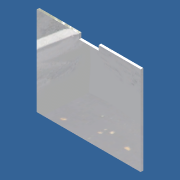
# Autodesk Inventor part: side panel for hinge
Saved by Autodesk Inventor 2012 (Build 160160000, 160)
## iProperties
Created: 2012-02-06
Part Number: side panel for hinge
Material: Default
Document SubType Name: Modeling
Designer: Allison Garza
Density: 1 g/cm^3
Author: Allison Garza
Autodesk Inventor part; units mm, degrees
ref_plane "YZ Plane" through (0, 0, 0) normal (1, 0, 0) x (0, 1, 0)
ref_plane "XZ Plane" through (0, 0, 0) normal (0, 1, 0) x (-1, 0, 0)
ref_plane "XY Plane" through (0, 0, 0) normal (0, 0, 1) x (1, 0, 0)
sketch "Sketch1" plane through (0, 0, 0) normal (0, 0, 1) x (1, 0, 0)
  line L0 (-13.9496, 17.395) -> (119.4004, 17.395)
  line L1 (119.4004, 17.395) -> (119.4004, -96.905)
  line L2 (119.4004, -96.905) -> (-13.9496, -96.905)
  line L3 (-13.9496, -96.905) -> (-13.9496, 17.395)
  point P0 (0, 0)
  dimension "d0" = 133.35
  dimension "d1" = 114.3
  constraints: 8 end point, 2 parallel, 1 horizontal, 1 perpendicular
  measures "d0" distance of L0.start L0.end
  measures "d1" distance of L2.end L0.start
extrude "Extrusion1" add sketch "Sketch1" along normal blind 3.175
sketch "Sketch2" plane through (0, 0, 3.175) normal (0, 0, 1) x (1, 0, 0)
  line L0 (-13.9496, 17.395) -> (119.4004, 17.395) projected
  line L1 (40.0254, 17.395) -> (65.4254, 17.395)
  line L2 (65.4254, 17.395) -> (65.4254, 11.045)
  line L3 (65.4254, 11.045) -> (40.0254, 11.045)
  line L4 (40.0254, 11.045) -> (40.0254, 17.395)
  point P0 (0, 0)
  dimension "d4" = 6.35
  dimension "d5" = 25.4
  dimension "d6" = 53.975
  constraints: 8 end point, 2 parallel, 1 horizontal, 1 perpendicular, 1 point on line
  measures "d4" distance of L1.end L2.end
  measures "d5" distance of L2.end L3.end
  measures "d6" distance of L0.start L1.start
extrude "Extrusion2" cut sketch "Sketch2" against normal blind 3.175
body "Solid1"
